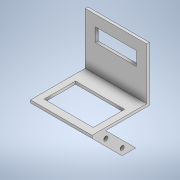
# Autodesk Inventor part: Subj_Cam
Saved by Autodesk Inventor 2021 (Build 250183000, 183)
## iProperties
Created: 2021-05-09
Part Number: Subj_Cam
Material: Genérico
Document SubType Name: Modeling
Designer: Marc
Density: 1 g/cm^3
Appearance: Valor por defecto
Author: Marc
## iProperties of the stored document _3DPrint.ipt
Created: 2021-05-09
Part Number: _3DPrint
Material: Genérico
Document SubType Name: Modeling
Designer: Marc
Density: 1 g/cm^3
Appearance: Valor por defecto
Author: Marc
Autodesk Inventor part; units mm, degrees
ref_plane "YZ Plane" through (0, 0, 0) normal (1, 0, 0) x (0, 1, 0)
ref_plane "XZ Plane" through (0, 0, 0) normal (0, 1, 0) x (-1, 0, 0)
ref_plane "XY Plane" through (0, 0, 0) normal (0, 0, 1) x (1, 0, 0)
sketch "Boceto1" plane through (0, 0, 0) normal (0, 0, 1) x (1, 0, 0)
  line L0 (-22.5, 19.94) -> (22.5, 19.94)
  line L1 (22.5, 19.94) -> (22.5, -20.06)
  line L2 (22.5, -20.06) -> (-22.5, -20.06)
  line L3 (-22.5, -20.06) -> (-22.5, 19.94)
  line L4 (0, 19.94) -> (0, 11.94)
  line L5 (15, 12.06) -> (-15, 12.06)
  line L6 (-15, 12.06) -> (-15, 2.06)
  line L7 (-15, 2.06) -> (15, 2.06)
  line L8 (15, 2.06) -> (15, 12.06)
  point P0 (0, 0)
  dimension "d0" = 45
  dimension "d1" = 40
  dimension "d2" = 8
  dimension "d4" = 30
  dimension "d5" = 10
  constraints: 18 end point, 4 perpendicular, 2 parallel, 1 horizontal, 1 midpoint, 1 vertical
  measures "d0" distance of L1.end L2.end
  measures "d1" distance of L0.end L1.end
  measures "d2" distance of L4.start L4.end
  measures "d4" distance of L5.start L5.end
  measures "d5" distance of L5.end L6.end
extrude "Extrusión1" add sketch "Boceto1" along normal blind 2
sketch "Boceto2" plane through (0, 0, 2) normal (0, 0, 1) x (1, 0, 0)
  line L0 (-22.5, 19.94) -> (-22.5, -20.06) projected
  line L1 (-22.5, -20.06) -> (22.5, -20.06)
  line L2 (22.5, -20.06) -> (22.5, -18.06)
  line L3 (22.5, -18.06) -> (-22.5, -18.06)
  line L4 (-22.5, -18.06) -> (-22.5, -20.06)
  point P0 (0, 0)
  dimension "d8" = 45
  dimension "d9" = 2
  constraints: 8 end point, 2 parallel, 1 horizontal, 1 perpendicular
  measures "d8" distance of L3.end L2.end
  measures "d9" distance of L2.end L1.end
extrude "Extrusión2" add sketch "Boceto2" along normal blind 40
sketch "Boceto3" plane through (-22.5, -18.06, 2) normal (0, 1, 0) x (1, 0, 0)
  line L0 (22.5, -34.62) -> (4.5, -34.62)
  line L1 (4.5, -34.62) -> (4.5, -11.62)
  line L2 (4.5, -11.62) -> (40.5, -11.62)
  line L3 (40.5, -11.62) -> (40.5, -34.62)
  line L4 (40.5, -34.62) -> (22.5, -34.62)
  point P0 (22.5, 2)
  dimension "d15" = 23
  dimension "d16" = 36
  constraints: 10 end point, 4 perpendicular, 1 horizontal, 1 point on line
  measures "d15" distance of L0.end L1.end
  measures "d16" distance of L1.end L2.end
extrude "Extrusión3" cut sketch "Boceto3" against normal blind 2
sketch "Boceto4" plane through (22.5, -20.06, 0) normal (1, 0, 0) x (0, 0, -1)
  line L0 (-20, -22) -> (-42, 0)
  line L1 (-20, -22) -> (-10, -22)
  line L2 (-10, -22) -> (-32, 0)
  line L3 (-42, 0) -> (-32, 0)
  point P0 (0, 20.06)
  dimension "d38" = 10
  constraints: 8 end point
  measures "d38" distance of L0.start L1.end
extrude "Extrusión4" add sketch "Boceto4" against normal blind 2
sketch "Boceto6" plane through (22.5, 19.94, 2) normal (1, 0, 0) x (0, 0, -1)
  line L0 (-40, -40) -> (-40, -45)
  circle A0 centre (-30, -45) radius 1.5
  circle A1 centre (-18, -57) radius 1.5
  point P0 (2, -19.94)
  dimension "d31" = 5
  constraints: 2 centre point, 2 end point, 1 vertical
  measures "d31" distance of L0.start L0.end
extrude "Extrusión6" cut sketch "Boceto6" against normal blind 2
sketch "Boceto7" plane through (0, 0, 42) normal (0, 0, 1) x (1, 0, 0)
  line L0 (-22.5, -20.06) -> (20.5, -20.06) projected
  line L1 (20.5, -20.06) -> (18, -20.06)
  line L2 (18, -20.06) -> (18, -22.56)
  line L3 (18, -22.56) -> (20.5, -22.56)
  line L4 (20.5, -20.06) -> (20.5, -42.06) projected
  line L5 (20.5, -20.06) -> (20.5, -22.56)
  point P0 (0, 0)
  dimension "d39" = 2.5
  dimension "d40" = 2.5
  constraints: 8 end point, 3 perpendicular, 2 point on line
  measures "d39" distance of L0.end L1.end
  measures "d40" distance of L1.end L2.end
extrude "Extrusión7" add sketch "Boceto7" against normal blind 12.5
sketch "Boceto9" plane through (20.5, -22.56, 42) normal (1, 0, 0) x (0, 0, -1)
  line L0 (22, -19.5) -> (2.5, 0) projected
  line L1 (0, 2.5) -> (0, 0) projected
  line L2 (2.5, 0) -> (0, 0)
  line L3 (0, 0) -> (0, 2.5)
  line L4 (0, 2.5) -> (2.5, 0)
  line L5 (0, 2.5) -> (22, -19.5) projected
  point P0 (42, 22.56)
  constraints: 6 end point, 2 collinear, 1 perpendicular
extrude "Extrusión8" cut sketch "Boceto9" against normal blind 12
sketch "Boceto10" plane through (20.5, -22.56, 29.5) normal (1, 0, 0) x (0, 0, -1)
  line L0 (-2.5, 2.5) -> (0, 2.5) projected
  line L1 (0, 0) -> (0, 2.5)
  line L2 (-2.5, 2.5) -> (0, 0) projected
  line L3 (0, 2.5) -> (-2.5, 2.5)
  line L4 (-2.5, 2.5) -> (0, 0)
  point P0 (29.5, 22.56)
  constraints: 6 end point, 1 collinear, 1 perpendicular, 1 vertical
extrude "Extrusión9" cut sketch "Boceto10" against normal blind 12
